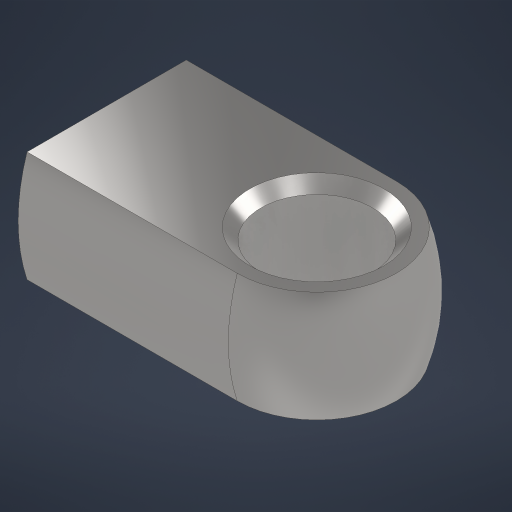
# Autodesk Inventor part: GMW-6-1 eye M6x1
Saved by Autodesk Inventor 2023 (Build 270158000, 158)
## iProperties
Created: 2023-03-02
Part Number: GMW-6-1 eye M6x1
Material: Steel, Alloy
Document SubType Name: Modeling
Designer: roota
Density: 7.73 g/cm^3
Appearance: Semi-Polished
Author: roota
Autodesk Inventor part; units mm, degrees
ref_plane "YZ Plane" through (0, 0, 0) normal (1, 0, 0) x (0, 1, 0)
ref_plane "XZ Plane" through (0, 0, 0) normal (0, 1, 0) x (-1, 0, 0)
ref_plane "XY Plane" through (0, 0, 0) normal (0, 0, 1) x (1, 0, 0)
sketch "Sketch1" plane through (0, 0, 0) normal (0, 0, 1) x (1, 0, 0)
  line L0 (0, 0) -> (27, 0)
  line L1 (27, 0) -> (27, 10)
  line L2 (27, 10) -> (0, 10)
  line L3 (0, 10) -> (0, 0)
  dimension "d0" = 27
  dimension "d1" = 10
  constraints: 8 end point, 2 parallel, 1 horizontal, 1 perpendicular
  measures "d0" distance of L2.end L1.end
  measures "d1" distance of L1.end L0.end
extrude "Extrusion1" add sketch "Sketch1" along normal blind 16
fillet "Fillet1" radius 8 2 edges at (27, 5, 16) (27, 5, 0)
sketch "Sketch2" plane through (0, 10, 16) normal (0, 1, 0) x (1, 0, 0)
  circle A0 centre (19, 8) radius 5.05
  arc A1 (19, 0) -> (19, 16) centre (19, 8) ccw projected
  point P0 (0, 16)
  dimension "d5" = 10.1
  constraints: 1 centre point, 1 concentric
  measures "d5" diameter of A0
extrude "Extrusion2" cut sketch "Sketch2" against normal through all
sketch "Sketch3" plane through (0, 0, 0) normal (-1, 0, 0) x (0, 0, 1)
  line L0 (0, 0) -> (16, 10) construction
  point P0 (8, 5)
  point P1 (8, 5)
  constraints: 2 end point, 1 coincident, 1 midpoint
hole "Hole1" at (0, 5, 8) direction (1, 0, 0) diameter 4.917 depth 12 tip angle 118
sketch "Sketch4" plane through (0, 0, 0) normal (-1, 0, 0) x (0, 0, 1)
  line L0 (0, 0) -> (16, 0) projected
  arc A0 (15.1987, 0) -> (15.1987, 10) centre (0, 5) ccw
  line L1 (0, 10) -> (16, 10) projected
  line L2 (16, 10) -> (16, 0) projected
  point P0 (16, 5)
  dimension "d15" = 16
  constraints: 2 point on circle, 2 point on line, 1 centre point, 1 tangent, 1 vertical alignment
  measures "d15" radius of A0
sketch3d "3D Sketch1"
  line L0 (0, 10, 16) -> (19, 10, 16)
  arc A0 (19, 10, 0) -> (24.6569, 10, 2.3431) centre (19, 10, 8) ccw
  arc A1 (24.6569, 10, 2.3431) -> (27, 10, 8) centre (19, 10, 8) ccw
  arc A2 (27, 10, 8) -> (24.6569, 10, 13.6569) centre (19, 10, 8) ccw
  arc A3 (24.6569, 10, 13.6569) -> (19, 10, 16) centre (19, 10, 8) ccw
  line L1 (19, 10, 0) -> (0, 10, 0)
sweep "Sweep1" cut profiles "Sketch4" path "3D Sketch1"
chamfer "Chamfer1" distance 1 angle 45 3 edges at (13.95, 10, 8) (13.95, 0, 8) (0, 5, 5.5415)
body "Solid1"
